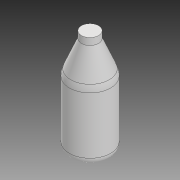
# Autodesk Inventor part: 2L bottle
Saved by Autodesk Inventor 2020 (Build 240168000, 168)
## iProperties
Created: 2021-05-05
Part Number: 2L bottle
Material: Generic
Document SubType Name: Modeling
Designer: DDeGo
Density: 1 g/cm^3
Appearance: Default
Author: DDeGo
Autodesk Inventor part; units mm, degrees
ref_plane "YZ Plane" through (0, 0, 0) normal (1, 0, 0) x (0, 1, 0)
ref_plane "XZ Plane" through (0, 0, 0) normal (0, 1, 0) x (-1, 0, 0)
ref_plane "XY Plane" through (0, 0, 0) normal (0, 0, 1) x (1, 0, 0)
sketch "Sketch1" plane through (0, 0, 0) normal (0, 0, 1) x (1, 0, 0)
  line L0 (0, 0) -> (35, 0)
  line L1 (55, 20) -> (55, 120) construction
  line L2 (52.2444, 206.3696) -> (25, 285)
  line L3 (25, 285) -> (25, 305)
  line L4 (25, 305) -> (0, 305)
  line L5 (0, 305) -> (0, 0)
  arc A0 (55, 190) -> (52.2444, 206.3696) centre (5, 190) ccw
  arc A1 (35, 0) -> (55, 20) centre (35, 20) ccw
  line L6 (55, 120) -> (50, 106.3786)
  line L7 (50, 106.3786) -> (50, 33.6214)
  line L8 (50, 33.6214) -> (55, 20)
  line L9 (55, 120) -> (55, 190)
  point P0 (55, 0)
  dimension "d1" = 55
  dimension "d4" = 50
  dimension "d6" = 25
  dimension "d7" = 20
  dimension "d8" = 115
  dimension "d9" = 20
  dimension "d10" = 70
  dimension "d11" = 120
  dimension "d12" = 5
  constraints: 20 end point, 6 tangent, 4 perpendicular, 4 point on circle, 2 centre point, 2 parallel, 2 point on line, 1 equal length, 1 horizontal, 1 vertical
  measures "d1" distance between parallel lines of L1 L5
  measures "d4" radius of A0
  measures "d6" distance between parallel lines of L5 L3
  measures "d7" radius of A1
  measures "d8" distance from line of L9.end L4
  measures "d9" distance of L2.end L3.end
  measures "d10" distance of L1.end L9.end
  measures "d11" distance from line of L0 L1.end
  measures "d12" distance between parallel lines of L1 L7
revolve "Revolution1" add sketch "Sketch1" angle 360 about axis through (0, 305, 0) along (0, -1, 0)
body "Solid1"
